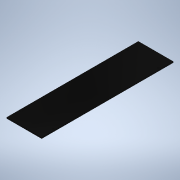
# Autodesk Inventor part: 三段目アクリル板
Saved by Autodesk Inventor 2022 (Build 260153000, 153)
## iProperties
Created: 2022-12-07
Part Number: 三段目アクリル板
Material: ABS プラスチック
Document SubType Name: Modeling
Designer: tdn82
Density: 1.06 g/cm^3
Appearance: 光沢 - 黒
Author: tdn82
Autodesk Inventor part; units mm, degrees
ref_plane "YZ Plane" through (0, 0, 0) normal (1, 0, 0) x (0, 1, 0)
ref_plane "XZ Plane" through (0, 0, 0) normal (0, 1, 0) x (-1, 0, 0)
ref_plane "XY Plane" through (0, 0, 0) normal (0, 0, 1) x (1, 0, 0)
sketch "スケッチ1" plane through (0, 0, 0) normal (0, 1, 0) x (-1, 0, 0)
  line L0 (0, 0) -> (-53, 0)
  line L1 (-53, 0) -> (-53, -200)
  line L2 (-53, -200) -> (0, -200)
  line L3 (0, -200) -> (0, 0)
  dimension "d0" = 200
  dimension "d1" = 53
  constraints: 8 end point, 2 parallel, 1 horizontal, 1 perpendicular
  measures "d0" distance of L2.end L0.start
  measures "d1" distance of L0.start L0.end
extrude "押し出し1" add sketch "スケッチ1" along normal blind 2
sketch "スケッチ3" plane through (0, 0, 0) normal (0, -1, 0) x (1, 0, 0)
  line L0 (53, 0) -> (53, -200) projected
  line L1 (53, -200) -> (0, -200) projected
  point P0 (0, 0)
  point P1 (50.5, -20)
  point P2 (50.5, -180)
  point P3 (3, -180)
  point P4 (3, -20)
  dimension "d4" = 2.5
  dimension "d5" = 180
  dimension "d6" = 160
  measures "d4" distance from line of point (50.5, -20) L0
  measures "d5" distance from line of point (50.5, -20) L1
  measures "d6" distance of point (50.5, -180) point (50.5, -20)
hole "穴1" at (50.5, 0, -20) at (50.5, 0, -180) at (3, 0, -180) at (3, 0, -20) direction (0, 1, 0) diameter 3 end through all
